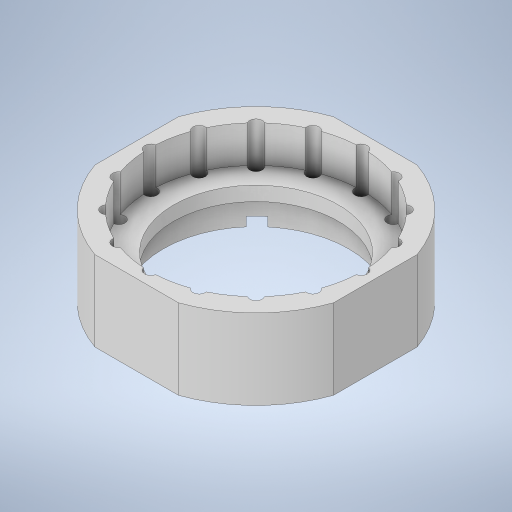
# Autodesk Inventor part: 사이클로이드 기어 하우징
Saved by Autodesk Inventor 2023 (Build 270158000, 158)
## iProperties
Created: 2022-06-19
Part Number: 사이클로이드 기어 하우징
Material: 일반
Document SubType Name: Modeling
Designer: fly01
Density: 1 g/cm^3
Appearance: 기본값
Author: fly01
Autodesk Inventor part; units mm, degrees
ref_plane "YZ Plane" through (0, 0, 0) normal (1, 0, 0) x (0, 1, 0)
ref_plane "XZ Plane" through (0, 0, 0) normal (0, 1, 0) x (-1, 0, 0)
ref_plane "XY Plane" through (0, 0, 0) normal (0, 0, 1) x (1, 0, 0)
sketch "스케치1" plane through (0, 0, 0) normal (0, 0, 1) x (1, 0, 0)
  line L0 (-25, -30) -> (25, -30) construction
  line L1 (30, -25) -> (30, 25) construction
  line L2 (25, 30) -> (-25, 30) construction
  line L3 (-30, 25) -> (-30, -25) construction
  line L4 (-30, -30) -> (30, 30) construction
  line L5 (30, -30) -> (-30, 30) construction
  arc A0 (-25, 30) -> (-30, 25) centre (-25, 25) ccw
  arc A1 (30, 25) -> (25, 30) centre (25, 25) ccw
  arc A2 (25, -30) -> (30, -25) centre (25, -25) ccw
  arc A3 (-30, -25) -> (-25, -30) centre (-25, -25) ccw
  circle A4 centre (0, 0) radius 7.5
  circle A5 centre (0, 0) radius 35 construction
  circle A6 centre (-24.7487, 24.7487) radius 2
  circle A7 centre (-24.7487, -24.7487) radius 2
  circle A8 centre (24.7487, -24.7487) radius 2
  circle A9 centre (24.7487, 24.7487) radius 2
  circle A10 centre (0, 0) radius 32.6
  circle A11 centre (0, 0) radius 25 construction
  line L6 (-25, 40) -> (25, 40)
  arc A12 (40, 25) -> (25, 40) centre (25, 25) ccw
  line L7 (40, 25) -> (40, -25)
  arc A13 (25, -40) -> (40, -25) centre (25, -25) ccw
  line L8 (25, -40) -> (-25, -40)
  arc A14 (-40, -25) -> (-25, -40) centre (-25, -25) ccw
  line L9 (-40, -25) -> (-40, 25)
  arc A15 (-25, 40) -> (-40, 25) centre (-25, 25) ccw
  dimension "d4" = 70
  dimension "d0" = 60
  dimension "d1" = 60
  dimension "d2" = 5
  dimension "d3" = 15
  dimension "d5" = 4
  dimension "d8" = 360
  dimension "d10" = 65.2
  dimension "d11" = 50
  dimension "d12" = 10
  constraints: 20 end point, 16 point on circle, 15 centre point, 9 point on line, 8 tangent, 4 coincident, 4 parallel, 3 equal radius, 2 midpoint, 2 perpendicular, 1 horizontal, 19 other
  measures "d0" distance of L5.end L4.end
  measures "d1" distance of L4.end L5.start
  measures "d2" radius of A0
  measures "d3" diameter of A4
  measures "d5" diameter of A6
  measures "d10" diameter of A10
  measures "d11" diameter of A11
  measures "d12" distance between parallel lines of L2 L6
extrude "돌출1" add sketch "스케치1" along normal blind 10.2 contours L6 A12 L7 A13 L8 A14 L9 A15
sketch "스케치2" plane through (0, 0, 0) normal (0, 0, -1) x (-1, 0, 0)
  line L0 (25, -40) -> (-25, -40) projected
  arc A0 (25, -40) -> (40, -25) centre (25, -25) ccw projected
  line L1 (40, 25) -> (40, -25) projected
  arc A1 (40, 25) -> (25, 40) centre (25, 25) ccw projected
  line L2 (-25, 40) -> (25, 40) projected
  arc A2 (-25, 40) -> (-40, 25) centre (-25, 25) ccw projected
  line L3 (-40, -25) -> (-40, 25) projected
  arc A3 (-40, -25) -> (-25, -40) centre (-25, -25) ccw projected
  circle A4 centre (0, 0) radius 32.6 construction
  circle A5 centre (-24.7487, 24.7487) radius 2 projected
  circle A6 centre (-24.7487, -24.7487) radius 2 projected
  circle A7 centre (24.7487, -24.7487) radius 2 projected
  circle A8 centre (24.7487, 24.7487) radius 2 projected
  circle A9 centre (0, 0) radius 29
  dimension "d15" = 58
  constraints: 1 centre point, 1 coincident
  measures "d15" diameter of A9
extrude "돌출2" add sketch "스케치2" along normal blind 5 contours L0 A3 L3 A2 L2 A1 L1 A0 | A5 | A6 | A7 | A8
sketch "스케치10" plane through (0, 0, -5) normal (0, 0, -1) x (-1, 0, 0)
  circle A0 centre (0, 0) radius 35 construction
  circle A1 centre (0, -37) radius 2 construction
  circle A2 centre (0, -37) radius 2.2
  dimension "d30" = 70
  dimension "d31" = 4
  dimension "d32" = 0.2
  constraints: 3 centre point, 1 coincident, 1 tangent
  measures "d30" diameter of A0
  measures "d31" diameter of A1
  measures "d32" radial gap between concentric circles of A1 A2
extrude "돌출5" cut sketch "스케치10" against normal blind 4
pattern_circular "원형 패턴1" count 16 over 360 about axis through (0, 0, 0) along (0, 0, -1) of "돌출5"
sketch "스케치11" plane through (0, 0, -5) normal (0, 0, -1) x (-1, 0, 0)
  circle A0 centre (0, -37) radius 2.2 projected
  circle A1 centre (0, 0) radius 37.5
  circle A2 centre (-26.163, 26.163) radius 2.2 projected
  circle A3 centre (-14.1593, 34.1835) radius 2.2 projected
  circle A4 centre (0, 37) radius 2.2 projected
  circle A5 centre (14.1593, 34.1835) radius 2.2 projected
  circle A6 centre (26.163, 26.163) radius 2.2 projected
  circle A7 centre (34.1835, 14.1593) radius 2.2 projected
  circle A8 centre (37, 0) radius 2.2 projected
  circle A9 centre (34.1835, -14.1593) radius 2.2 projected
  circle A10 centre (26.163, -26.163) radius 2.2 projected
  circle A11 centre (14.1593, -34.1835) radius 2.2 projected
  circle A12 centre (0, -37) radius 2.2 projected
  line L0 (25, 40) -> (-25, 40) projected
  arc A13 (-25, 40) -> (-40, 25) centre (-25, 25) ccw projected
  line L1 (-40, 25) -> (-40, -25) projected
  arc A14 (-40, -25) -> (-25, -40) centre (-25, -25) ccw projected
  line L2 (-25, -40) -> (25, -40) projected
  arc A15 (25, -40) -> (40, -25) centre (25, -25) ccw projected
  line L3 (40, -25) -> (40, 25) projected
  arc A16 (40, 25) -> (25, 40) centre (25, 25) ccw projected
  circle A17 centre (0, 0) radius 29 projected
  circle A18 centre (-14.1593, -34.1835) radius 2.2 projected
  circle A19 centre (-26.163, -26.163) radius 2.2 projected
  circle A20 centre (-34.1835, -14.1593) radius 2.2 projected
  circle A21 centre (-37, 0) radius 2.2 projected
  circle A22 centre (-34.1835, 14.1593) radius 2.2 projected
  point P0 (16.3187, -33.7631)
  point P1 (12.335, -35.4132)
  point P2 (2.156, -37.438)
  point P3 (-2.156, -37.438)
  point P4 (-27.9971, 24.9481)
  point P5 (-24.9481, 27.9971)
  point P6 (-16.3187, 33.7631)
  point P7 (-12.335, 35.4132)
  point P8 (-2.156, 37.438)
  point P9 (2.156, 37.438)
  point P10 (12.335, 35.4132)
  point P11 (16.3187, 33.7631)
  point P12 (24.9481, 27.9971)
  point P13 (27.9971, 24.9481)
  point P14 (33.7631, 16.3187)
  point P15 (35.4132, 12.335)
  point P16 (37.438, -2.156)
  point P17 (37.438, 2.156)
  point P18 (35.4132, -12.335)
  point P19 (33.7631, -16.3187)
  point P20 (27.9971, -24.9481)
  point P21 (24.9481, -27.9971)
  point P22 (-35.4132, 12.335)
  point P23 (-33.7631, 16.3187)
  point P24 (-12.335, -35.4132)
  point P25 (-16.3187, -33.7631)
  point P26 (-24.9481, -27.9971)
  point P27 (-27.9971, -24.9481)
  point P28 (-33.7631, -16.3187)
  point P29 (-35.4132, -12.335)
  point P30 (-37.438, -2.156)
  point P31 (-37.438, 2.156)
  dimension "d38" = 75
  constraints: 1 coincident, 2 other
extrude "돌출6" add sketch "스케치11" along normal blind 13 contours A16 L3 A15 L2 A14 L1 A13 L0
sketch "스케치13" plane through (0, 0, 10.2) normal (0, 0, 1) x (1, 0, 0)
  circle A0 centre (-24.7487, -24.7487) radius 2 projected
  circle A1 centre (-24.7487, -24.7487) radius 2 projected
  line L0 (-28.7902, -24.7487) -> (-26.7695, -21.2487)
  line L1 (-26.7695, -21.2487) -> (-22.728, -21.2487)
  line L2 (-22.728, -21.2487) -> (-20.7073, -24.7487)
  line L3 (-20.7073, -24.7487) -> (-22.728, -28.2487)
  line L4 (-22.728, -28.2487) -> (-26.7695, -28.2487)
  line L5 (-26.7695, -28.2487) -> (-28.7902, -24.7487)
  line L6 (0, 0) -> (-8.2451, 0)
  line L7 (0, 0) -> (0, 11.1173)
  circle A2 centre (-24.7487, 24.7487) radius 2
  circle A3 centre (-24.7487, 24.7487) radius 2
  line L8 (-28.7902, 24.7487) -> (-26.7695, 21.2487)
  line L9 (-26.7695, 21.2487) -> (-22.728, 21.2487)
  line L10 (-22.728, 21.2487) -> (-20.7073, 24.7487)
  line L11 (-20.7073, 24.7487) -> (-22.728, 28.2487)
  line L12 (-22.728, 28.2487) -> (-26.7695, 28.2487)
  line L13 (-26.7695, 28.2487) -> (-28.7902, 24.7487)
  circle A4 centre (24.7487, -24.7487) radius 2
  circle A5 centre (24.7487, -24.7487) radius 2
  line L14 (28.7902, -24.7487) -> (26.7695, -21.2487)
  line L15 (26.7695, -21.2487) -> (22.728, -21.2487)
  line L16 (22.728, -21.2487) -> (20.7073, -24.7487)
  line L17 (20.7073, -24.7487) -> (22.728, -28.2487)
  line L18 (22.728, -28.2487) -> (26.7695, -28.2487)
  line L19 (26.7695, -28.2487) -> (28.7902, -24.7487)
  circle A6 centre (24.7487, 24.7487) radius 2
  circle A7 centre (24.7487, 24.7487) radius 2
  line L20 (28.7902, 24.7487) -> (26.7695, 21.2487)
  line L21 (26.7695, 21.2487) -> (22.728, 21.2487)
  line L22 (22.728, 21.2487) -> (20.7073, 24.7487)
  line L23 (20.7073, 24.7487) -> (22.728, 28.2487)
  line L24 (22.728, 28.2487) -> (26.7695, 28.2487)
  line L25 (26.7695, 28.2487) -> (28.7902, 24.7487)
  line L26 (-26.7695, -21.2487) -> (-25.2227, -18.5697)
  line L27 (-25.2227, -18.5697) -> (-22.728, -21.2487)
  line L28 (-26.7695, 21.2487) -> (-24.7487, 17.7487)
  line L29 (-24.7487, 17.7487) -> (-22.728, 21.2487)
  line L30 (26.7695, -21.2487) -> (24.7487, -17.7487)
  line L31 (24.7487, -17.7487) -> (22.728, -21.2487)
  line L32 (26.7695, 21.2487) -> (24.7487, 17.7487)
  line L33 (24.7487, 17.7487) -> (22.728, 21.2487)
  dimension "d41" = 7
  constraints: 68 end point, 27 symmetric about line, 6 centre point, 4 coincident, 4 parallel, 1 horizontal, 1 vertical, 19 other
  measures "d41" distance between parallel lines of L4 L1
extrude "돌출7" cut sketch "스케치13" against normal blind 3.2 contours A0 | L0 L1 L2 L3 L4 L5 | L13 L12 L11 L10 L9 L8 | L19 L18 L17 L16 L15 L14 | L20 L21 L22 L23 L24 L25
sketch "스케치15" plane through (0, 0, 10.2) normal (0, 0, 1) x (1, 0, 0)
  circle A0 centre (0, 0) radius 42.5
  circle A1 centre (0, 0) radius 58.6603
  dimension "d49" = 85
  constraints: 2 centre point, 2 coincident
  measures "d49" diameter of A0
extrude "돌출9" cut sketch "스케치15" against normal blind 114.25
sketch "스케치16" plane through (0, 0, 10.2) normal (0, 0, 1) x (1, 0, 0)
  line L0 (37.3094, 12) -> (36.1547, 10)
  line L1 (36.1547, 10) -> (33.8453, 10)
  line L2 (33.8453, 10) -> (32.6906, 12)
  line L3 (32.6906, 12) -> (33.8453, 14)
  line L4 (33.8453, 14) -> (36.1547, 14)
  line L5 (36.1547, 14) -> (37.3094, 12)
  circle A0 centre (35, 12) radius 1.15
  line L6 (0, 0) -> (45.2961, 0)
  line L7 (40, -14.3614) -> (40, 14.3614) projected
  line L8 (37.3094, -12) -> (36.1547, -10)
  line L9 (36.1547, -10) -> (33.8453, -10)
  line L10 (33.8453, -10) -> (32.6906, -12)
  line L11 (32.6906, -12) -> (33.8453, -14)
  line L12 (33.8453, -14) -> (36.1547, -14)
  line L13 (36.1547, -14) -> (37.3094, -12)
  circle A1 centre (35, -12) radius 1.15
  dimension "d52" = 4
  dimension "d53" = 2.3
  dimension "d64" = 12
  dimension "d65" = 35
  constraints: 26 end point, 8 symmetric about line, 2 centre point, 2 coincident, 2 horizontal, 14 other
  measures "d52" distance between parallel lines of L1 L4
  measures "d53" diameter of A0
  measures "d64" distance from line of L6 point (35, 12)
  measures "d65" horizontal distance of L6.start point (35, 12)
extrude "돌출11" cut sketch "스케치16" against normal blind 6 contours A0 | A1
pattern_circular "원형 패턴2" count 4 over 360 about axis through (0, 0, 0) along (0, 0, 1) of "돌출11"
sketch "스케치17" plane through (0, 0, -18) normal (0, 0, -1) x (-1, 0, 0)
  arc A0 (-40, -14.3614) -> (-14.3614, -40) centre (0, 0) ccw projected
  line L0 (-14.3614, -40) -> (14.3614, -40) projected
  arc A1 (14.3614, -40) -> (40, -14.3614) centre (0, 0) ccw projected
  line L1 (40, -14.3614) -> (40, 14.3614) projected
  arc A2 (40, 14.3614) -> (14.3614, 40) centre (0, 0) ccw projected
  line L2 (14.3614, 40) -> (-14.3614, 40) projected
  arc A3 (-14.3614, 40) -> (-40, 14.3614) centre (0, 0) ccw projected
  line L3 (-40, 14.3614) -> (-40, -14.3614) projected
  arc A4 (-33.7631, 16.3187) -> (-35.4132, 12.335) centre (-34.1835, 14.1593) ccw projected
  arc A5 (-27.9971, 24.9481) -> (-33.7631, 16.3187) centre (0, 0) ccw projected
  arc A6 (-24.9481, 27.9971) -> (-27.9971, 24.9481) centre (-26.163, 26.163) ccw projected
  arc A7 (-16.3187, 33.7631) -> (-24.9481, 27.9971) centre (0, 0) ccw projected
  arc A8 (-12.335, 35.4132) -> (-16.3187, 33.7631) centre (-14.1593, 34.1835) ccw projected
  arc A9 (-2.156, 37.438) -> (-12.335, 35.4132) centre (0, 0) ccw projected
  arc A10 (2.156, 37.438) -> (-2.156, 37.438) centre (0, 37) ccw projected
  arc A11 (12.335, 35.4132) -> (2.156, 37.438) centre (0, 0) ccw projected
  arc A12 (16.3187, 33.7631) -> (12.335, 35.4132) centre (14.1593, 34.1835) ccw projected
  arc A13 (24.9481, 27.9971) -> (16.3187, 33.7631) centre (0, 0) ccw projected
  arc A14 (27.9971, 24.9481) -> (24.9481, 27.9971) centre (26.163, 26.163) ccw projected
  arc A15 (33.7631, 16.3187) -> (27.9971, 24.9481) centre (0, 0) ccw projected
  arc A16 (35.4132, 12.335) -> (33.7631, 16.3187) centre (34.1835, 14.1593) ccw projected
  arc A17 (37.438, 2.156) -> (35.4132, 12.335) centre (0, 0) ccw projected
  arc A18 (37.438, -2.156) -> (37.438, 2.156) centre (37, 0) ccw projected
  arc A19 (35.4132, -12.335) -> (37.438, -2.156) centre (0, 0) ccw projected
  arc A20 (33.7631, -16.3187) -> (35.4132, -12.335) centre (34.1835, -14.1593) ccw projected
  arc A21 (27.9971, -24.9481) -> (33.7631, -16.3187) centre (0, 0) ccw projected
  arc A22 (24.9481, -27.9971) -> (27.9971, -24.9481) centre (26.163, -26.163) ccw projected
  arc A23 (16.3187, -33.7631) -> (24.9481, -27.9971) centre (0, 0) ccw projected
  arc A24 (12.335, -35.4132) -> (16.3187, -33.7631) centre (14.1593, -34.1835) ccw projected
  arc A25 (2.156, -37.438) -> (12.335, -35.4132) centre (0, 0) ccw projected
  arc A26 (-2.156, -37.438) -> (2.156, -37.438) centre (0, -37) ccw projected
  arc A27 (-12.335, -35.4132) -> (-2.156, -37.438) centre (0, 0) ccw projected
  arc A28 (-16.3187, -33.7631) -> (-12.335, -35.4132) centre (-14.1593, -34.1835) ccw projected
  arc A29 (-24.9481, -27.9971) -> (-16.3187, -33.7631) centre (0, 0) ccw projected
  arc A30 (-27.9971, -24.9481) -> (-24.9481, -27.9971) centre (-26.163, -26.163) ccw projected
  arc A31 (-33.7631, -16.3187) -> (-27.9971, -24.9481) centre (0, 0) ccw projected
  arc A32 (-35.4132, -12.335) -> (-33.7631, -16.3187) centre (-34.1835, -14.1593) ccw projected
  arc A33 (-37.438, -2.156) -> (-35.4132, -12.335) centre (0, 0) ccw projected
  arc A34 (-37.438, 2.156) -> (-37.438, -2.156) centre (-37, 0) ccw projected
  arc A35 (-35.4132, 12.335) -> (-37.438, 2.156) centre (0, 0) ccw projected
  arc A36 (14.7054, -42) -> (42, -14.7054) centre (0, 0) ccw
  line L4 (14.7054, -42) -> (-14.7054, -42)
  arc A37 (-42, -14.7054) -> (-14.7054, -42) centre (0, 0) ccw
  line L5 (-42, -14.7054) -> (-42, 14.7054)
  arc A38 (-14.7054, 42) -> (-42, 14.7054) centre (0, 0) ccw
  line L6 (-14.7054, 42) -> (14.7054, 42)
  arc A39 (42, 14.7054) -> (14.7054, 42) centre (0, 0) ccw
  line L7 (42, 14.7054) -> (42, -14.7054)
  dimension "d66" = 2
  constraints: 8 end point, 8 point on circle, 4 centre point, 7 other
  measures "d66" radial gap between concentric circles of A1 A36
extrude "돌출12" add sketch "스케치17" against normal up to surface (28.2 mm away) contours L4 A37 L5 A38 L6 A39 L7 A36
